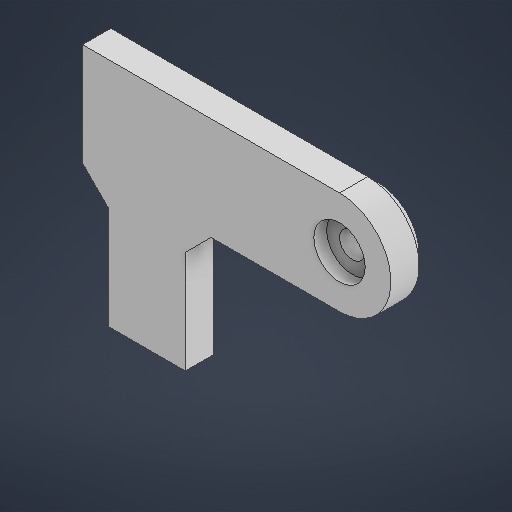
# Autodesk Inventor part: belt_leg
Saved by Autodesk Inventor 2025.1 (Build 291241000, 241)
## iProperties
Created: 2024-12-12
Part Number: belt_leg
Material: Všeobecné
Document SubType Name: Modeling
Designer: lukas
Density: 1 g/cm^3
Appearance: Výchozí
Author: lukas
Autodesk Inventor part; units mm, degrees
ref_plane "YZ Plane" through (0, 0, 0) normal (1, 0, 0) x (0, 1, 0)
ref_plane "XZ Plane" through (0, 0, 0) normal (0, 1, 0) x (-1, 0, 0)
ref_plane "XY Plane" through (0, 0, 0) normal (0, 0, 1) x (1, 0, 0)
sketch "Náčrt1" plane through (0, 0, 0) normal (0, 0, 1) x (1, 0, 0)
  line L0 (-74, 0) -> (94, 0) projected
  line L1 (0, 63) -> (0, -63) projected
  line L2 (-40, -45) -> (-10, -45)
  line L3 (-10, -45) -> (-10, 5)
  line L4 (-10, 5) -> (50, 5)
  line L5 (50, 5) -> (50, 45)
  line L6 (50, 45) -> (-50, 45)
  line L7 (-50, 45) -> (-50, 5)
  line L8 (-50, 5) -> (-40, 5)
  line L9 (-40, 5) -> (-40, -45)
  circle A0 centre (50, 25) radius 20
  point P0 (0, 0)
  dimension "d0" = 100
  dimension "d1" = 40
  dimension "d2" = 40
  dimension "d3" = 10
  dimension "d4" = 30
  dimension "d5" = 50
  constraints: 16 end point, 6 perpendicular, 1 horizontal, 1 midpoint, 1 vertical, 5 other
  measures "d0" distance of L5.end L6.end
  measures "d1" distance of L4.end L5.end
  measures "d2" distance of L6.end L7.end
  measures "d3" distance of L7.end L8.end
  measures "d4" distance of L2.start L2.end
  measures "d5" distance of L2.end L3.end
extrude "Vysunutí1" add sketch "Náčrt1" along normal blind 15 contours L9 L8 L7 L6 L1 L4 L3 L0 | L0 L3 L2 L9 | L1 L6 A0 L4 | A0 L5 | L5 A0
sketch "Náčrt2" plane through (0, 0, 15) normal (0, 0, 1) x (1, 0, 0)
  arc A0 (50, 5) -> (50, 45) centre (50, 25) ccw projected
  line L0 (-40, 5) -> (-40, -45) projected
  line L1 (-40, -45) -> (-10, -45) projected
  line L2 (-10, -45) -> (-10, 5) projected
  line L3 (-10, 5) -> (50, 5) projected
  arc A1 (50, 5) -> (50, 45) centre (50, 25) ccw projected
  line L4 (50, 45) -> (-50, 45) projected
  line L5 (-50, 45) -> (-50, 5) projected
  line L6 (-50, 5) -> (-40, 5) projected
  line L7 (-74, 0) -> (94, 0) projected
  line L8 (0, 63) -> (0, -63) projected
  point P0 (0, 0)
  constraints: 1 coincident
hole "Díra1" at (50, 25, 15) direction (0, 0, -1) diameter 10 end through all counterbore diameter 20 counterbore depth 5
chamfer "Zkosení1" distance 4 angle 45 8 edges at (0, 45, 0) (70, 25, 0) (20, 5, 0) (-50, 25, 0) (-40, -20, 0) (-45, 5, 0) (-10, -20, 0) (-25, -45, 0)
ref_plane "Pracovní rovina1" through (0, 0, 7.5) normal (0, 0, 1) x (1, 0, 0)
sketch "Náčrt3" plane through (0, 0, 7.5) normal (0, 0, 1) x (1, 0, 0)
  circle A0 centre (50, 25) radius 10 projected
  line L0 (-40, 5) -> (-40, -45) projected
  line L1 (-40, -45) -> (-10, -45) projected
  line L2 (-10, -45) -> (-10, 5) projected
  line L3 (-10, 5) -> (50, 5) projected
  arc A1 (50, 5) -> (50, 45) centre (50, 25) ccw projected
  line L4 (50, 45) -> (-50, 45) projected
  line L5 (-50, 45) -> (-50, 5) projected
  line L6 (-50, 5) -> (-40, 5) projected
  line L7 (0, 5) -> (-10, -5)
  line L8 (0, 5) -> (4.4525, 5) construction
  point P0 (0, 0)
  dimension "d18" = 135
  dimension "d19" = 10
  constraints: 4 end point, 2 point on line, 1 horizontal
  measures "d18" angle of L7 L8
  measures "d19" horizontal distance of L7.start L7.end
extrude "Žebro1" add sketch "Náčrt3" along normal mid plane 7 rib yes fills toward (-5.0354, 0.0354) open curves L7
sketch "Náčrt4" plane through (-10, 5, 11) normal (0, 0, 1) x (1, 0, 0)
  line L0 (0, 0) -> (10, 0) projected
  line L1 (0, -10) -> (0, 0) projected
  line L2 (10, 0) -> (0, -10) projected
  line L3 (10, 0) -> (0, 0)
  line L4 (10, 0) -> (0, -10) projected
  line L5 (0, -10) -> (10, 0)
  point P0 (10, -5)
  constraints: 4 end point, 2 collinear
extrude "Vysunutí2" add sketch "Náčrt4" along normal blind 4
sketch "Náčrt5" plane through (0, 0, 7.5) normal (0, 0, 1) x (1, 0, 0)
  circle A0 centre (50, 25) radius 10 projected
  line L0 (-40, 5) -> (-40, -45) projected
  line L1 (-40, -45) -> (-10, -45) projected
  line L2 (-10, -45) -> (-10, -5) projected
  line L3 (-10, -5) -> (0, 5) projected
  line L4 (0, 5) -> (50, 5) projected
  arc A1 (50, 5) -> (50, 45) centre (50, 25) ccw projected
  line L5 (50, 45) -> (-50, 45) projected
  line L6 (-50, 45) -> (-50, 5) projected
  line L7 (-50, 5) -> (-40, 5) projected
  line L8 (-50, 5) -> (-40, -5)
  line L9 (-50, 5) -> (-38.3899, 5) construction
  point P0 (0, 0)
  dimension "d28" = 45
  dimension "d29" = 10
  constraints: 4 end point, 2 point on line, 1 horizontal
  measures "d28" angle of L8 L9
  measures "d29" horizontal distance of L8.start L8.end
extrude "Žebro2" add sketch "Náčrt5" along normal mid plane 7 rib yes fills toward (-44.9646, 0.0354) open curves L8
sketch "Náčrt6" plane through (-50, 5, 11) normal (0, 0, 1) x (1, 0, 0)
  line L0 (10, 0) -> (10, -10) projected
  line L1 (0, 0) -> (10, 0) projected
  line L2 (10, -10) -> (0, 0) projected
  line L3 (10, 0) -> (10, -50) projected
  line L4 (0, 0) -> (10, 0)
  line L5 (10, 0) -> (10, -10)
  point P0 (50, -5)
  constraints: 4 end point, 2 point on line, 1 collinear
extrude "Vysunutí3" add sketch "Náčrt6" along normal blind 4
